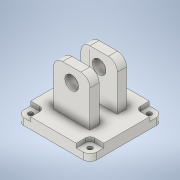
# Autodesk Inventor part: Befestigungsflansch
Saved by Autodesk Inventor 2020.3 (Build 243373000, 373)
## iProperties
Created: 2021-05-20
Part Number: Befestigungsflansch
Material: Stahl AISI 4130
Document SubType Name: Modeling
Designer: Preuß P. Ch.
Density: 7.85 g/cm^3
Appearance: Stahl
Author: Preuß P. Ch.
Autodesk Inventor part; units mm, degrees
ref_plane "YZ Plane" through (0, 0, 0) normal (1, 0, 0) x (0, 1, 0)
ref_plane "XZ Plane" through (0, 0, 0) normal (0, 1, 0) x (-1, 0, 0)
ref_plane "XY Plane" through (0, 0, 0) normal (0, 0, 1) x (1, 0, 0)
sketch "Skizze1" plane through (0, 0, 0) normal (0, 0, 1) x (1, 0, 0)
  line L0 (0, 80) -> (24, 80)
  line L1 (24, 80) -> (24, -80)
  line L2 (24, -80) -> (0, -80)
  line L3 (0, -80) -> (0, 80)
  line L4 (24, 40) -> (124, 40)
  line L5 (124, 40) -> (124, -40)
  line L6 (124, -40) -> (24, -40)
  line L7 (24, -40) -> (24, 40)
  point P0 (0, 0)
  point P1 (24, 0)
  point P2 (0, 0)
  point P3 (94, 0)
  point P4 (124, 0)
  dimension "d0" = 160
  dimension "d1" = 24
  dimension "d2" = 124
  dimension "d3" = 80
  dimension "d4" = 94
  constraints: 16 end point, 4 midpoint, 4 parallel, 2 horizontal, 2 perpendicular, 1 coincident, 1 horizontal alignment
  measures "d0" distance of L2.end L0.start
  measures "d1" distance of L1.end L2.end
  measures "d2" distance between parallel lines of L5 L3
  measures "d3" distance of L4.end L5.end
  measures "d4" distance from line of point (94, 0) L3
extrude "Extrusion1" add sketch "Skizze1" along normal mid plane 160 contours L0 L1 L2 L3
extrude "Extrusion2" add sketch "Skizze1" along normal mid plane 80 contours L4 L5 L6 L1
extrude "Extrusion3" cut sketch "Skizze1" along normal mid plane 40 contours L4 L5 L6 L1
fillet "Rundung1" radius 20 4 edges at (124, 40, 30) (124, 40, -30) (124, -40, -30) (124, -40, 30)
hole "Bohrung1" at (94, 0, 0) direction (0, 0, -1) diameter 30 end through all both
sketch "Skizze2" plane through (24, -80, 80) normal (1, 0, 0) x (0, 0, -1)
  line L0 (0, 160) -> (30, 160)
  line L1 (30, 160) -> (30, 130)
  line L2 (30, 130) -> (0, 130)
  line L3 (0, 130) -> (0, 160)
  point P0 (80, 80)
  dimension "d19" = 30
  dimension "d20" = 30
  constraints: 8 end point, 2 parallel, 1 horizontal, 1 perpendicular
  measures "d19" distance of L1.end L2.end
  measures "d20" distance of L0.end L1.end
extrude "Extrusion4" cut sketch "Skizze2" against normal blind 9
pattern_circular "Runde Anordnung1" count 4 over 360 about axis through (-10, 0, 0) along (1, 0, 0) of "Extrusion4"
sketch "Skizze3" plane through (24, 50, 50) normal (1, 0, 0) x (0, 0, -1)
  line L0 (-15, 15) -> (115, 15)
  line L1 (115, 15) -> (115, -115)
  line L2 (115, -115) -> (-15, -115)
  line L3 (-15, -115) -> (-15, 15)
  line L4 (-15, 15) -> (115, -115) construction
  line L5 (115, 15) -> (-15, -115) construction
  point P0 (50, -50)
  dimension "d26" = 130
  dimension "d27" = 130
  constraints: 12 end point, 2 midpoint, 2 parallel, 1 horizontal, 1 perpendicular
  measures "d26" distance of L1.end L2.end
  measures "d27" distance of L0.end L1.end
hole "Bohrung2" at (24, 65, 65) at (24, -65, 65) at (24, 65, -65) at (24, -65, -65) direction (-1, 0, 0) diameter 10.5 end through all
fillet "Rundung2" radius 15 4 edges at (7.5, 80, -80) (7.5, -80, -80) (7.5, -80, 80) (7.5, 80, 80)
fillet "Rundung3" radius 10 4 edges at (19.5, -50, 50) (19.5, -50, -50) (19.5, 50, -50) (19.5, 50, 50)
equation "\"d5\" = d0"
